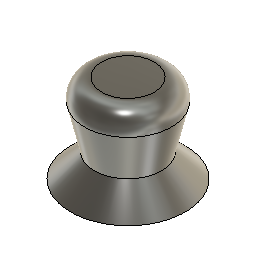
joystiick (Autodesk Fusion 360 design; units mm, degrees)
Autodesk Fusion 360 part; units mm, degrees
note: some values were not read from the file. Set by a fixed rule: which sketch regions a step uses.
sketch "Sketch1" plane through (0, 0, 0) normal (0, 0, 1) x (1, 0, 0)
  circle A0 centre (0, 0) radius 3.8
extrude "Extrude1" add sketch "Sketch1" along normal blind 10
sketch "Sketch2" plane through (0, 0, 0) normal (0, 0, -1) x (1, 0, 0)
  circle A0 centre (0, 0) radius 3.8
  line L0 (1.15, 1.15) -> (-1.15, 1.15)
  line L1 (-1.15, 1.15) -> (-1.15, -1.15)
  line L2 (-1.15, -1.15) -> (1.15, -1.15)
  line L3 (1.15, -1.15) -> (1.15, 1.15)
  line L4 (1.15, 1.15) -> (-1.15, -1.15) construction
  line L5 (-1.15, 1.15) -> (1.15, -1.15) construction
  dimension "d3" = 2.3
  dimension "d4" = 2.3
  constraint horizontal L0
  constraint perpendicular L0 L1
  constraint parallel L0 L2
  constraint parallel L1 L3
  constraint coincident L4 A0.centre
  constraint coincident L5 A0.centre
  constraint coincident A0.centre origin
  measures "d3" distance of L1.end L2.end
  measures "d4" distance of L0.end L1.end
sketch "Sketch3" plane through (0, 0, 0) normal (0, 0, -1) x (1, 0, 0)
  circle A0 centre (0, 0) radius 3.8
  circle A1 centre (0, 0) radius 6.5
  dimension "d7" = 13
  constraint coincident A0.centre A1.centre
  measures "d7" diameter of A1
extrude "Extrude3" add sketch "Sketch3" against normal blind 2.7
chamfer "Chamfer1" distance 2.7 angle 45 1 edges at (-6.0601, -2.3505, 2.7)
sketch "Sketch4" plane through (0, 0, 0) normal (0, 0, -1) x (1, 0, 0)
  circle A0 centre (0, 0) radius 6.5
  circle A1 centre (0, 0) radius 2.25
  dimension "d11" = 4.5
  constraint coincident A0.centre A1.centre
  measures "d11" diameter of A1
extrude "Extrude4" cut sketch "Sketch4" against normal blind 0.5 contours A1
extrude "Extrude5" cut 1 faces at (1.4364, 1.4089, 10) along direction (0, 0, -1) blind 7.3
extrude "Extrude6" add 1 faces at (-0.9575, 0.0466, 2.7) along direction (0, 0, 1) blind 7.3 draft 13
fillet "Fillet1" radius 2 1 edges at (-5.1141, 1.9836, 10)
sketch "Sketch5" plane through (0, 0, 0.5) normal (0, 0, -1) x (1, 0, 0)
  circle A0 centre (0, 0) radius 2.25
  line L0 (1.115, 1.115) -> (-1.115, 1.115)
  line L1 (-1.115, 1.115) -> (-1.115, -1.115)
  line L2 (-1.115, -1.115) -> (1.115, -1.115)
  line L3 (1.115, -1.115) -> (1.115, 1.115)
  line L4 (1.115, 1.115) -> (-1.115, -1.115) construction
  line L5 (-1.115, 1.115) -> (1.115, -1.115) construction
  dimension "d20" = 2.23
  dimension "d21" = 2.23
  constraint horizontal L0
  constraint perpendicular L0 L1
  constraint parallel L0 L2
  constraint parallel L1 L3
  constraint coincident L4 A0.centre
  constraint coincident L5 A0.centre
  constraint coincident A0.centre origin
  measures "d20" distance of L1.end L2.end
  measures "d21" distance of L0.end L1.end
extrude "Extrude7" cut sketch "Sketch5" against normal blind 2 contours L0 L1 L2 L3
extrude "Extrude8" cut 1 faces at (-1.4933, 0, 0.5) along direction (0, 0, 1) blind 0.25
